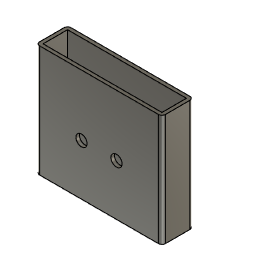
desk-phone-mount v4 (Autodesk Fusion 360 design; units mm, degrees)
Autodesk Fusion 360 part; units mm, degrees
sketch "front-mount" plane through (0, 0, 0) normal (0, 1, 0) x (1, 0, 0)
  line L0 (0, 0) -> (50, 0)
  line L1 (50, 0) -> (50, -19.25)
  line L2 (50, -19.25) -> (0, -19.25)
  line L3 (0, -19.25) -> (0, 0)
  line L4 (0, -19.25) -> (0, -23.25)
  line L5 (0, -23.25) -> (50, -23.25)
  line L6 (50, -23.25) -> (50, -19.25)
  line L7 (25, -19.25) -> (25, 0) construction
  line L8 (0, -9.625) -> (25, -9.625) construction
  circle A0 centre (12.5, -9.625) radius 1.625
  circle A1 centre (12.5, -9.625) radius 2.875
  circle A2 centre (37.5, -9.625) radius 2.875
  circle A3 centre (37.5, -9.625) radius 1.625
  circle A4 centre (12.5, -9.625) radius 4
  circle A5 centre (37.5, -9.625) radius 4
  dimension "d8" = 50
  dimension "d9" = 19.25
  dimension "d10" = 4
  dimension "d11" = 3.25
  dimension "d12" = 5.75
  dimension "d28" = 8
  constraint horizontal L0
  constraint vertical L1
  constraint horizontal L2
  constraint vertical L3
  constraint coincident L0.start L3.end
  constraint perpendicular L2 L4
  constraint perpendicular L4 L5
  constraint equal L4 L6
  constraint midpoint L2 L7.start
  constraint midpoint L0 L7.end
  constraint midpoint L3 L8.start
  constraint midpoint L7 L8.end
  constraint midpoint L8 A0.centre
  constraint concentric A0 A1
  constraint symmetric L7 A0 A3
  constraint symmetric L7 A1 A2
  constraint concentric A0 A4
  constraint symmetric L7 A4 A5
  measures "d8" distance of L0.start L0.end
  measures "d9" distance of L0.start L2.end
  measures "d10" distance of L2.end L4.end
  measures "d11" diameter of A0
  measures "d12" diameter of A1
  measures "d28" diameter of A4
extrude "Extrude1" add sketch "front-mount" along normal blind 4 contours L0 L1 L2 L3 | L2 L4 L5 L6 | A0 | A1 | A2 | A3 | A4 | A5 makes body 1
extrude "Extrude2" add sketch "front-mount" along normal blind 15 from surface at 4 contours L2 L4 L5 L6 bodies 1
sketch "Sketch3" plane through (0, 0, 23.25) normal (0, 0, 1) x (-1, 0, 0)
  line L0 (0, 0) -> (-50, 0)
  line L1 (-50, 0) -> (-50, -19)
  line L2 (-50, -19) -> (0, -19)
  line L3 (0, -19) -> (0, 0)
  line L4 (-50, -4) -> (0, -4)
  line L5 (0, 0) -> (-50, 0)
  line L6 (-50, 0) -> (-50, -4)
  line L7 (0, 0) -> (0, -4)
  line L8 (17.5, 20) -> (-67.5, 20)
  line L9 (-67.5, 20) -> (-67.5, 2.5)
  line L10 (-67.5, 2.5) -> (17.5, 2.5)
  line L11 (17.5, 2.5) -> (17.5, 20)
  line L12 (-25, -4) -> (-25, 0) construction
  line L13 (-70, 22.5) -> (-70, 0)
  line L14 (-70, 0) -> (20, 0)
  line L15 (20, 0) -> (20, 22.5)
  line L16 (20, 22.5) -> (-70, 22.5)
  line L17 (-25, 22.5) -> (-25, 0) construction
  point P0 (-25, 0)
  dimension "d18" = 17.5
  dimension "d19" = 85
  dimension "d20" = 2.5
  constraint horizontal L8
  constraint vertical L9
  constraint horizontal L10
  constraint vertical L11
  constraint midpoint L4 L12.start
  constraint midpoint L5 P0
  constraint midpoint L16 L17.start
  constraint midpoint L14 P0
  constraint coincident P0 L12.end
  measures "d18" distance of L8.start L10.end
  measures "d19" distance of L8.start L8.end
extrude "Extrude3" add sketch "Sketch3" along normal blind 30 separate body contours L0 L5 L13 L14 L15 L16 makes body 2
extrude "Extrude4" add sketch "Sketch3" against normal blind 50 contours L0 L5 L13 L14 L15 L16 bodies 2
extrude "Extrude5" add sketch "Sketch3" along normal blind 3 from surface at -50 contours L8 L9 L10 L11 bodies 1 2
extrude "Extrude6" cut sketch "front-mount" against normal up to surface (22.5 mm away) contours A0 | A1 | A2 | A3 | A4 | A5 bodies 2
extrude "Extrude7" cut sketch "front-mount" along normal up to surface (4 mm away) contours A0 | A3 bodies 1
extrude "Extrude8" cut sketch "front-mount" along normal blind 2.25 contours A1 | A2 bodies 1
fillet "Fillet1" radius 3 5 edges at (0, 19, 21.25) (50, 19, 21.25) (50, 0, 9.625) (50, 0, 21.25) (0, 0, 11.625) on bodies 1
fillet "Fillet2" radius 2.5 4 edges at (-20, -22.5, 13.25) (-20, 0, 13.25) (70, -22.5, 13.25) (70, 0, 13.25) on bodies 2
sketch "Sketch4" plane through (0, 0, 23.25) normal (0, 0, 1) x (-1, 0, 0)
  arc A0 (0, -3) -> (-3, 0) centre (-3, -3) ccw
  line L0 (-3, 0) -> (-47, 0)
  arc A1 (-47, 0) -> (-50, -3) centre (-47, -3) ccw
  line L1 (-50, -3) -> (-50, -16)
  arc A2 (-50, -16) -> (-47, -19) centre (-47, -16) ccw
  line L2 (-47, -19) -> (-3, -19)
  arc A3 (-3, -19) -> (0, -16) centre (-3, -16) ccw
  line L3 (0, -16) -> (0, -3)
  line L4 (-25, -19) -> (-25, 0) construction
  line L5 (-50, -9.5) -> (-25, -9.5) construction
  circle A4 centre (-25, -9.5) radius 1.5
  circle A5 centre (-25, -9.5) radius 2.875
  dimension "d39" = 3
  dimension "d40" = 5.75
  constraint midpoint L2 L4.start
  constraint midpoint L0 L4.end
  constraint midpoint L1 L5.start
  constraint midpoint L4 L5.end
  constraint coincident L5.end A4.centre
  constraint concentric A4 A5
  measures "d39" diameter of A4
  measures "d40" diameter of A5
extrude "Extrude9" cut sketch "Sketch4" against normal up to surface (4 mm away) contours A4 bodies 1
extrude "Extrude10" cut sketch "Sketch4" against normal blind 1.75 contours A5 bodies 1
extrude "Extrude11" add sketch "front-mount" against normal up to surface (2.5 mm away) contours A1 | A2 | A4 | A5 bodies 2
named bodies: "phone-mount", "phone-holder"
